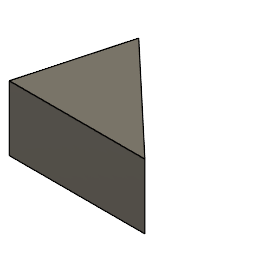
replay (Autodesk Fusion 360 design; units mm, degrees)
Autodesk Fusion 360 part; units mm, degrees
ref_plane "工作平面1" through (0, -2, 0) normal (0, 1, 0) x (0, 0, 1)
sketch "草图1" plane through (0, -2, 0) normal (0, 1, 0) x (1, 0, 0)
  line L0 (49, -45) -> (14, -12)
  line L1 (14, -12) -> (5, -45)
  line L2 (5, -45) -> (49, -45)
extrude "拉伸1" add sketch "草图1" along normal blind 21
